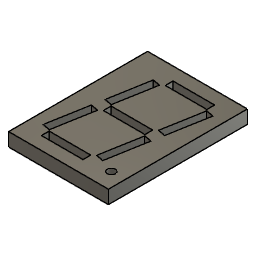
LED_NEON_7SEG (Autodesk Fusion 360 design; units mm, degrees)
Autodesk Fusion 360 part; units mm, degrees
note: some values were not read from the file. Set by a fixed rule: the direction of a hole.
sketch "Sketch1" plane through (0, 0, 0) normal (0, 1, 0) x (1, 0, 0)
  line L0 (0, 0) -> (67.2, 0)
  line L1 (67.2, 0) -> (67.2, 93.6)
  line L2 (67.2, 93.6) -> (0, 93.6)
  line L3 (0, 93.6) -> (0, 0)
  line L4 (33.6, 0) -> (33.6, 93.6) construction
  line L5 (25.3479, 0) -> (41.8521, 93.6) construction
  line L6 (21.8513, 82.2531) -> (57.8513, 82.2531) construction
  line L7 (9.3487, 11.3469) -> (45.3487, 11.3469) construction
  line L8 (27.3487, 11.3469) -> (39.8513, 82.2531) construction
  line L9 (9.3487, 11.3469) -> (21.8513, 82.2531) construction
  line L10 (45.3487, 11.3469) -> (57.8513, 82.2531) construction
  line L11 (25.8513, 84.8531) -> (53.8513, 84.8531)
  line L12 (53.8513, 84.8531) -> (53.8513, 79.6531)
  line L13 (53.8513, 79.6531) -> (25.8513, 79.6531)
  line L14 (25.8513, 79.6531) -> (25.8513, 84.8531)
  line L15 (39.8513, 84.8531) -> (39.8513, 79.6531) construction
  line L16 (15.6, 46.8) -> (51.6, 46.8) construction
  line L17 (18.7257, 64.5265) -> (12.4743, 29.0735) construction
  line L18 (48.4743, 29.0735) -> (54.7257, 64.5265) construction
  line L19 (18.5962, 78.7653) -> (13.7341, 51.1907)
  line L20 (13.7341, 51.1907) -> (18.8551, 50.2877)
  line L21 (18.8551, 50.2877) -> (23.7172, 77.8624)
  line L22 (23.7172, 77.8624) -> (18.5962, 78.7653)
  line L23 (21.2862, 64.0751) -> (16.1652, 64.978) construction
  line L24 (13.3487, 13.9469) -> (41.3487, 13.9469)
  line L25 (41.3487, 13.9469) -> (41.3487, 8.7469)
  line L26 (41.3487, 8.7469) -> (13.3487, 8.7469)
  line L27 (13.3487, 8.7469) -> (13.3487, 13.9469)
  line L28 (27.3487, 8.7469) -> (27.3487, 13.9469) construction
  line L29 (19.6, 49.4) -> (47.6, 49.4)
  line L30 (47.6, 49.4) -> (47.6, 44.2)
  line L31 (47.6, 44.2) -> (19.6, 44.2)
  line L32 (19.6, 44.2) -> (19.6, 49.4)
  line L33 (33.6, 44.2) -> (33.6, 49.4) construction
  line L34 (54.5962, 78.7653) -> (59.7172, 77.8624)
  line L35 (59.7172, 77.8624) -> (54.8551, 50.2877)
  line L36 (54.8551, 50.2877) -> (49.7341, 51.1907)
  line L37 (49.7341, 51.1907) -> (54.5962, 78.7653)
  line L38 (52.1652, 64.978) -> (57.2862, 64.0751) construction
  line L39 (12.3449, 43.3123) -> (17.4659, 42.4093)
  line L40 (17.4659, 42.4093) -> (12.6038, 14.8347)
  line L41 (12.6038, 14.8347) -> (7.4828, 15.7376)
  line L42 (7.4828, 15.7376) -> (12.3449, 43.3123)
  line L43 (15.0348, 28.622) -> (9.9138, 29.5249) construction
  line L44 (48.3449, 43.3123) -> (53.4659, 42.4093)
  line L45 (53.4659, 42.4093) -> (48.6038, 14.8347)
  line L46 (48.6038, 14.8347) -> (43.4828, 15.7376)
  line L47 (43.4828, 15.7376) -> (48.3449, 43.3123)
  line L48 (45.9138, 29.5249) -> (51.0348, 28.622) construction
  point P0 (39.8513, 82.2531)
  point P1 (27.3487, 11.3469)
  dimension "d1" = 93.6
  dimension "d2" = 10
  dimension "d3" = 36
  dimension "d4" = 72
  dimension "d5" = 28
  dimension "d6" = 5.2
  dimension "d7" = 36
  dimension "d22" = 67.2
  constraint horizontal L0
  constraint vertical L1
  constraint horizontal L2
  constraint vertical L3
  constraint coincident L0.start L3.end
  constraint midpoint L0 L4.start
  constraint midpoint L2 L4.end
  constraint coincident L0 L5.start
  constraint coincident L2 L5.end
  constraint midpoint L4 L5
  constraint perpendicular L4 L6
  constraint midpoint L6 P0
  constraint coincident L5 P0
  constraint perpendicular L1 L7
  constraint midpoint L7 P1
  constraint coincident L5 P1
  constraint equal L6 L7
  constraint coincident P1 L8.start
  constraint coincident P0 L8.end
  constraint midpoint L4 L8
  constraint horizontal L11
  constraint vertical L12
  constraint horizontal L13
  constraint vertical L14
  constraint midpoint L11 L15.start
  constraint midpoint L13 L15.end
  constraint midpoint P0 L15
  constraint midpoint L9 L16.start
  constraint midpoint L10 L16.end
  constraint coincident L9 L17.start
  constraint coincident L9 L17.end
  constraint parallel L9 L17
  constraint midpoint L9 L17
  constraint coincident L10 L18.start
  constraint coincident L10 L18.end
  constraint parallel L10 L18
  constraint equal L17 L18
  constraint midpoint L10 L18
  constraint perpendicular L17 L20
  constraint perpendicular L20 L21
  constraint perpendicular L19 L22
  constraint parallel L19 L21
  constraint midpoint L21 L23.start
  constraint midpoint L19 L23.end
  constraint perpendicular L19 L23
  constraint coincident L17.start L23
  constraint equal L14 L22
  constraint midpoint L17.start L23
  constraint equal L13 L21
  constraint horizontal L24
  constraint vertical L25
  constraint horizontal L26
  constraint vertical L27
  constraint midpoint L26 L28.start
  constraint midpoint L24 L28.end
  constraint midpoint P1 L28
  constraint equal L13 L24
  constraint equal L14 L27
  constraint horizontal L29
  constraint vertical L30
  constraint horizontal L31
  constraint vertical L32
  constraint midpoint L31 L33.start
  constraint midpoint L29 L33.end
  constraint midpoint L4 L33
  constraint equal L14 L32
  constraint equal L13 L29
  constraint perpendicular L10 L34
  constraint perpendicular L34 L35
  constraint perpendicular L10 L36
  constraint parallel L35 L37
  constraint midpoint L37 L38.start
  constraint midpoint L35 L38.end
  constraint midpoint L18.end L38
  constraint equal L13 L37
  constraint equal L14 L34
  constraint perpendicular L9 L39
  constraint perpendicular L39 L40
  constraint perpendicular L9 L41
  constraint parallel L40 L42
  constraint midpoint L40 L43.start
  constraint midpoint L42 L43.end
  constraint midpoint L17.end L43
  constraint equal L14 L39
  constraint equal L13 L42
  constraint perpendicular L18 L44
  constraint perpendicular L44 L45
  constraint perpendicular L10 L46
  constraint parallel L45 L47
  constraint midpoint L47 L48.start
  constraint midpoint L45 L48.end
  constraint midpoint L18.start L48
  constraint equal L14 L44
  constraint equal L13 L47
  measures "d1" distance of L0.end L1.end
  measures "d2" angle of L4 L5
  measures "d3" distance of L6.start L6.end
  measures "d4" distance of L6.end L7.end
  measures "d5" distance of L11.start L11.end
  measures "d6" distance of L11.start L13.end
  measures "d7" distance of L17.start L17.end
  measures "d22" distance of L1.end L2.end
extrude "Extrude1" add sketch "Sketch1" along normal blind 6
extrude "Extrude2" add sketch "Sketch1" against normal blind 3 contours L0 L1 L2 L3 | L11 L12 L13 L14 | L19 L20 L21 L22 | L24 L25 L26 L27 | L29 L30 L31 L32 | L34 L35 L36 L37 | L39 L40 L41 L42 | L44 L45 L46 L47
sketch "Sketch2" plane through (0, 0, 0) normal (0, 1, 0) x (1, 0, 0)
  line L0 (41.3487, 8.7469) -> (13.3487, 8.7469)
  line L1 (13.3487, 8.7469) -> (13.3487, 13.9469)
  line L2 (13.3487, 13.9469) -> (41.3487, 13.9469)
  line L3 (41.3487, 13.9469) -> (41.3487, 8.7469)
  line L4 (18.5962, 78.7653) -> (23.7172, 77.8624)
  line L5 (23.7172, 77.8624) -> (18.8551, 50.2877)
  line L6 (18.8551, 50.2877) -> (13.7341, 51.1907)
  line L7 (13.7341, 51.1907) -> (18.5962, 78.7653)
  line L8 (53.8513, 79.6531) -> (25.8513, 79.6531)
  line L9 (25.8513, 79.6531) -> (25.8513, 84.8531)
  line L10 (25.8513, 84.8531) -> (53.8513, 84.8531)
  line L11 (53.8513, 84.8531) -> (53.8513, 79.6531)
  line L12 (47.6, 44.2) -> (19.6, 44.2)
  line L13 (19.6, 44.2) -> (19.6, 49.4)
  line L14 (19.6, 49.4) -> (47.6, 49.4)
  line L15 (47.6, 49.4) -> (47.6, 44.2)
  line L16 (54.8551, 50.2877) -> (49.7341, 51.1907)
  line L17 (49.7341, 51.1907) -> (54.5962, 78.7653)
  line L18 (54.5962, 78.7653) -> (59.7172, 77.8624)
  line L19 (59.7172, 77.8624) -> (54.8551, 50.2877)
  line L20 (12.6038, 14.8347) -> (7.4828, 15.7376)
  line L21 (7.4828, 15.7376) -> (12.3449, 43.3123)
  line L22 (12.3449, 43.3123) -> (17.4659, 42.4093)
  line L23 (17.4659, 42.4093) -> (12.6038, 14.8347)
  line L24 (48.6038, 14.8347) -> (43.4828, 15.7376)
  line L25 (43.4828, 15.7376) -> (48.3449, 43.3123)
  line L26 (48.3449, 43.3123) -> (53.4659, 42.4093)
  line L27 (53.4659, 42.4093) -> (48.6038, 14.8347)
  line L28 (0, 93.6) -> (0, 0)
  line L29 (0, 0) -> (67.2, 0)
  line L30 (67.2, 0) -> (67.2, 93.6)
  line L31 (67.2, 93.6) -> (0, 93.6)
  line L32 (53.8513, 84.8531) -> (49.8513, 84.8531)
  line L33 (49.8513, 84.8531) -> (49.8513, 79.6531)
  line L34 (49.8513, 79.6531) -> (53.8513, 79.6531)
  line L35 (53.8513, 79.6531) -> (53.8513, 84.8531)
  line L36 (47.6, 49.4) -> (43.6, 49.4)
  line L37 (43.6, 49.4) -> (43.6, 44.2)
  line L38 (43.6, 44.2) -> (47.6, 44.2)
  line L39 (47.6, 44.2) -> (47.6, 49.4)
  line L40 (41.3487, 13.9469) -> (37.3487, 13.9469)
  line L41 (37.3487, 13.9469) -> (37.3487, 8.7469)
  line L42 (37.3487, 8.7469) -> (41.3487, 8.7469)
  line L43 (41.3487, 8.7469) -> (41.3487, 13.9469)
  line L44 (8.1774, 19.6769) -> (13.2984, 18.7739)
  line L45 (12.6038, 14.8347) -> (13.2984, 18.7739)
  line L46 (44.1774, 19.6769) -> (49.2984, 18.7739)
  line L47 (48.6038, 14.8347) -> (49.2984, 18.7739)
  line L48 (14.4287, 55.1299) -> (19.5497, 54.227)
  line L49 (18.8551, 50.2877) -> (19.5497, 54.227)
  line L50 (50.4287, 55.1299) -> (55.5497, 54.227)
  line L51 (55.5497, 54.227) -> (54.8551, 50.2877)
  line L52 (53.8513, 79.6531) -> (25.8513, 79.6531)
  line L53 (45.3487, 11.3469) -> (57.8513, 82.2531)
  line L54 (9.3487, 11.3469) -> (45.3487, 11.3469)
  line L55 (45.3487, 11.3469) -> (57.8513, 11.3469) construction
  line L56 (57.8513, 11.3469) -> (57.8513, 82.2531) construction
  dimension "d12" = 4
  constraint horizontal L32
  constraint vertical L33
  constraint horizontal L34
  constraint vertical L35
  constraint coincident L10.end L11.start
  constraint horizontal L36
  constraint vertical L37
  constraint horizontal L38
  constraint vertical L39
  constraint coincident L12 L37.end
  constraint coincident L14.end L15.start
  constraint horizontal L40
  constraint vertical L41
  constraint horizontal L42
  constraint vertical L43
  constraint coincident L0 L41.end
  constraint coincident L2.end L3.start
  constraint coincident L21 L44.start
  constraint coincident L23 L44.end
  constraint perpendicular L23 L44
  constraint coincident L20.start L23.end
  constraint perpendicular L44 L45
  constraint coincident L25 L46.start
  constraint coincident L27 L46.end
  constraint perpendicular L27 L46
  constraint coincident L24.start L27.end
  constraint perpendicular L46 L47
  constraint coincident L7 L48.start
  constraint coincident L5 L48.end
  constraint perpendicular L5 L48
  constraint coincident L5.end L6.start
  constraint perpendicular L48 L49
  constraint coincident L17 L50.start
  constraint coincident L19 L50.end
  constraint perpendicular L19 L50
  constraint coincident L16.start L19.end
  constraint perpendicular L16 L51
  constraint equal L32 L51
  constraint equal L32 L49
  constraint equal L32 L36
  constraint equal L32 L47
  constraint equal L32 L45
  constraint equal L32 L40
  constraint coincident L33.end L52
  constraint coincident L53.start L54.end
  constraint horizontal L55
  constraint coincident L53.end L56.end
  constraint vertical L56
  measures "d12" distance of L10.end L32.end
extrude "Extrude3" cut sketch "Sketch2" against normal up to surface (3 mm away) contours L0 L3 L41 L42 L43 L54 | L2 L3 L40 L41 L43 L54 | L5 L6 L7 L48 L49 | L8 L10 L11 L32 L33 L34 L35 L52 | L12 L14 L15 L36 L37 L38 L39 | L16 L19 L50 L51 L53 | L16 L17 L50 L53 | L20 L21 L23 L44 L45 | L24 L27 L46 L47 L53 | L24 L25 L46 L53
hole "Hole1" at (57.8513, 0, -11.3469) direction (0, -1, 0) diameter 5.4 depth 13 tip angle 180
hole "Hole2" at (57.8513, 0, -11.3469) direction (0, 1, 0) diameter 5.4 depth 13 tip angle 180
equation "d1 = d3 * 2.6"
equation "d4 = d3 * 2"
equation "d6 = 5 mm + ( 0.1 * 2 ) * 1 mm"
equation "d7 = d4 / 2"
equation "d22 = d5 * 2.4"
